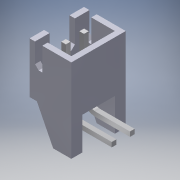
# Autodesk Inventor part: 4A-0363.43
Saved by Autodesk Inventor 2016 SP2 (Build 200236200, 236)
## iProperties
Created: 2016-11-21
Part Number: 4A-0363.43
Material: Plástico PPS
Document SubType Name: Modeling
Designer: laguerre
Density: 1.637 g/cm^3
Appearance: Blanco frío
Description: WAFER 2.5mm CRIMP STYLE CONNECTOR
Author: laguerre
Autodesk Inventor part; units mm, degrees
ref_plane "YZ Plane" through (0, 0, 0) normal (1, 0, 0) x (0, 1, 0)
ref_plane "XZ Plane" through (0, 0, 0) normal (0, 1, 0) x (-1, 0, 0)
sketch "Boceto40" plane through (0, 0, 0) normal (1, 0, 0) x (0, 1, 0)
  line L0 (0, 0) -> (0, 5.75)
  line L1 (0, 5.75) -> (-7, 5.75)
  line L2 (-7, 5.75) -> (-7, 4.75)
  line L3 (-7, 4.75) -> (-11.5, 2.5)
  line L4 (-11.5, 2.5) -> (-11.5, 0)
  line L5 (-11.5, 0) -> (0, 0)
  dimension "d374" = 5.75
  dimension "d375" = 7
  dimension "d376" = 2.5
  dimension "d377" = 4.5
  dimension "d378" = 1
  constraints: 12 end point, 2 perpendicular, 1 horizontal, 1 parallel, 1 vertical
  measures "d374" distance between parallel lines of L5 L1
  measures "d375" distance of L0.end L1.end
  measures "d376" distance of L3.end L4.end
  measures "d377" horizontal distance of L2.end L3.end
  measures "d378" distance of L1.end L2.end
extrude "Extrusión13" add sketch "Boceto40" along normal mid plane 7.5
sketch "Boceto41" plane through (0, 0, 0) normal (1, 0, 0) x (0, 1, 0)
  line L0 (0, 0) -> (0, 5.75) construction
  line L1 (0, 5.75) -> (-7, 5.75) construction
  line L2 (-7, 5.75) -> (-7, 4.75) construction
  line L3 (-7, 4.75) -> (-11.5, 2.5) construction
  line L4 (-11.5, 2.5) -> (-11.5, 0) construction
  line L5 (-11.5, 0) -> (0, 0) construction
  line L6 (0, 5) -> (-4.7, 5)
  line L7 (-4.7, 5) -> (-4.7, 2.5)
  line L8 (-4.7, 2.5) -> (-5, 2.2)
  line L9 (-5, 2.2) -> (-5, 0.75)
  line L10 (-5, 0.75) -> (0, 0.75)
  line L11 (0, 0.75) -> (0, 5)
  dimension "d381" = 0.75
  dimension "d382" = 0.75
  dimension "d383" = 4.7
  dimension "d384" = 5
  dimension "d385" = 2.5
  dimension "d386" = 45
  constraints: 12 end point, 3 perpendicular, 2 point on line, 1 horizontal, 1 parallel
  measures "d381" distance between parallel lines of L1 L6
  measures "d382" distance between parallel lines of L5 L10
  measures "d383" distance between parallel lines of L0 L7
  measures "d384" distance between parallel lines of L0 L9
  measures "d385" distance from line of L7.end L6
  measures "d386" angle of L9 L8
extrude "Extrusión14" cut sketch "Boceto41" along normal mid plane 6
sketch "Boceto42" plane through (0, 0, 0) normal (1, 0, 0) x (0, 1, 0)
  line L0 (0, 0) -> (0, 5.75) construction
  line L1 (0, 5.75) -> (-7, 5.75) construction
  line L2 (-7, 5.75) -> (-7, 4.75) construction
  line L3 (-7, 4.75) -> (-11.5, 2.5) construction
  line L4 (-11.5, 2.5) -> (-11.5, 0) construction
  line L5 (-11.5, 0) -> (0, 0) construction
  line L6 (0, 5) -> (-2.7, 5)
  line L7 (-3.2, 4.5) -> (-3.2, 4)
  line L8 (-3.2, 4) -> (0, 4)
  line L9 (0, 4) -> (0, 5)
  line L10 (-3.2, 4.5) -> (-2.7, 5)
  point P0 (-3.2, 5)
  dimension "d389" = 1
  dimension "d390" = 0.75
  dimension "d391" = 3.2
  dimension "d392" = 0.5
  dimension "d393" = 0.5
  constraints: 10 end point, 3 point on line, 2 parallel, 1 horizontal, 1 perpendicular
  measures "d389" distance between parallel lines of L6 L8
  measures "d390" distance between parallel lines of L1 L6
  measures "d391" distance between parallel lines of L0 L7
  measures "d392" distance of L7.start point (-3.2, 5)
  measures "d393" distance of L6.end point (-3.2, 5)
extrude "Extrusión15" cut sketch "Boceto42" along normal mid plane 10
sketch "Boceto43" plane through (-3.75, -7, 5.75) normal (0, 0, 1) x (1, 0, 0)
  line L0 (0, 0) -> (7.5, 0) construction
  line L1 (7.5, 7) -> (7.5, 0) construction
  line L2 (0, 7) -> (7.5, 7) construction
  line L3 (0, 0) -> (0, 7) construction
  line L4 (6, -4.7153) -> (1.5, -4.7153)
  line L5 (1.5, -4.7153) -> (1.5, 0)
  line L6 (1.5, 0) -> (6, 0)
  line L7 (6, 0) -> (6, -4.7153)
  point P0 (3.75, 7)
  dimension "d397" = 1.5
  dimension "d398" = 1.5
  constraints: 8 end point, 2 parallel, 1 horizontal, 1 perpendicular, 1 point on line
  measures "d397" distance between parallel lines of L5 L3
  measures "d398" distance between parallel lines of L1 L7
extrude "Extrusión16" cut sketch "Boceto43" against normal blind 10
ref_plane "Plano de trabajo12" through (-3, -0.4, 2.5) normal (0, 1, 0) x (1, 0, 0)
sketch "Boceto44" plane through (-3, -0.4, 2.5) normal (0, 1, 0) x (1, 0, 0)
  line L0 (0, 0) -> (6, 0) construction
  line L1 (0, 0) -> (0, -2.5) construction
  line L2 (0, -2.5) -> (6, -2.5) construction
  line L3 (6, -2.5) -> (6, 0) construction
  line L4 (4.57, -1.07) -> (3.93, -1.07)
  line L5 (3.93, -1.07) -> (3.93, -0.43)
  line L6 (3.93, -0.43) -> (4.57, -0.43)
  line L7 (4.57, -0.43) -> (4.57, -1.07)
  line L8 (2.07, -1.07) -> (1.43, -1.07)
  line L9 (1.43, -1.07) -> (1.43, -0.43)
  line L10 (1.43, -0.43) -> (2.07, -0.43)
  line L11 (2.07, -0.43) -> (2.07, -1.07)
  line L12 (3, 2.5) -> (3, -4.081) construction
  line L13 (4.25, -1.07) -> (4.25, -0.43) construction
  line L14 (1.75, -1.07) -> (1.75, -0.43) construction
  line L15 (4.57, -0.75) -> (3.93, -0.75) construction
  line L16 (2.07, -0.75) -> (1.43, -0.75) construction
  line L17 (-0.75, -3.25) -> (6.75, -3.25) projected
  dimension "d402" = 2.5
  dimension "d403" = 0.64
  dimension "d404" = 2.5
  constraints: 26 end point, 8 midpoint, 4 parallel, 3 equal length, 2 horizontal, 2 perpendicular, 1 point on line, 1 vertical, 1 other
  measures "d402" distance between parallel lines of L14 L13
  measures "d403" distance of L4.start L4.end
  measures "d404" distance between parallel lines of L15 L17
sketch "Boceto45" plane through (0, 0, 0) normal (1, 0, 0) x (0, 1, 0)
  line L0 (-0.4, 3.25) -> (-7.2, 3.25)
  line L1 (-9.2, 1.25) -> (-9.2, -3.4)
  line L2 (0, 0.75) -> (0, 4) projected
  arc A0 (-7.2, 3.25) -> (-9.2, 1.25) centre (-7.2, 1.25) ccw
  line L3 (0, 0) -> (-11.5, 0) projected
  dimension "d405" = 9.2
  dimension "d406" = 2
  dimension "d409" = 3.4
  constraints: 4 end point, 2 point on circle, 2 tangent, 1 centre point, 1 horizontal, 1 perpendicular
  measures "d405" distance between parallel lines of L1 L2
  measures "d406" radius of A0
  measures "d409" distance from line of L3 L1.end
sweep "Barrido1" add profiles "Boceto44" path "Boceto45" separate body path curves L0 A0 L1
sketch "Boceto46" plane through (-3.75, -7, 5.75) normal (0, 0, 1) x (1, 0, 0)
  line L0 (0, 0) -> (7.5, 0) construction
  line L1 (7.5, 7) -> (7.5, 0) construction
  line L2 (0, 7) -> (7.5, 7) construction
  line L3 (0, 0) -> (0, 7) construction
  line L4 (5.5, 7) -> (2, 7)
  line L5 (2, 7) -> (2, 3.9)
  line L6 (2.5, 3.4) -> (5, 3.4)
  line L7 (5.5, 3.9) -> (5.5, 7)
  line L8 (2, 3.9) -> (2.5, 3.4)
  line L9 (5.5, 3.9) -> (5, 3.4)
  point P0 (3.75, 7)
  point P1 (2, 3.4)
  point P2 (5.5, 3.4)
  dimension "d412" = 3.6
  dimension "d413" = 2
  dimension "d414" = 2
  dimension "d415" = 0.5
  dimension "d416" = 0.5
  dimension "d417" = 0.5
  dimension "d418" = 0.5
  constraints: 12 end point, 5 point on line, 2 parallel, 1 horizontal, 1 perpendicular
  measures "d412" distance between parallel lines of L2 L6
  measures "d413" distance between parallel lines of L3 L5
  measures "d414" distance between parallel lines of L1 L7
  measures "d415" distance of L5.end point (2, 3.4)
  measures "d416" distance of L6.start point (2, 3.4)
  measures "d417" distance of L7.start point (5.5, 3.4)
  measures "d418" distance of L6.end point (5.5, 3.4)
extrude "Extrusión17" cut sketch "Boceto46" against normal blind 1 bodies 1
